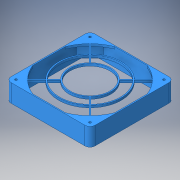
# Autodesk Inventor part: filterFrame
Saved by Autodesk Inventor 2016 (Build 200138000, 138)
## iProperties
Created: 2015-10-01
Part Number: filterFrame
Material: Generic
Document SubType Name: Modeling
Designer: xdlea
Density: 1 g/cm^3
Appearance: Cyan
fanCenter: 2.205 in
d39: 0.059 in
Author: xdlea
Autodesk Inventor part; units mm, degrees
ref_plane "YZ Plane" through (0, 0, 0) normal (1, 0, 0) x (0, 1, 0)
ref_plane "XZ Plane" through (0, 0, 0) normal (0, 1, 0) x (-1, 0, 0)
ref_plane "XY Plane" through (0, 0, 0) normal (0, 0, 1) x (1, 0, 0)
sketch "Sketch1" plane through (0, 0, 0) normal (0, 1, 0) x (-1, 0, 0)
  line L0 (-59.5, 59.5) -> (59.5, 59.5)
  line L1 (59.5, 59.5) -> (59.5, -59.5)
  line L2 (59.5, -59.5) -> (-59.5, -59.5)
  line L3 (-59.5, -59.5) -> (-59.5, 59.5)
  line L4 (-59.5, 59.5) -> (59.5, -59.5) construction
  line L5 (59.5, 59.5) -> (-59.5, -59.5) construction
  circle A0 centre (52.4, 52.4) radius 1.5
  circle A1 centre (52.4, -52.4) radius 1.5
  arc A2 (58, 23.2863) -> (23.2863, 58) centre (0, 0) ccw
  arc A3 (23.2863, -58) -> (58, -23.2863) centre (0, 0) ccw
  arc A4 (-58, -23.2863) -> (-23.2863, -58) centre (0, 0) ccw
  arc A5 (-23.2863, 58) -> (-58, 23.2863) centre (0, 0) ccw
  line L6 (23.2863, 58) -> (-23.2863, 58)
  line L7 (-58, 23.2863) -> (-58, -23.2863)
  line L8 (-23.2863, -58) -> (23.2863, -58)
  line L9 (58, -23.2863) -> (58, 23.2863)
  arc A6 (59.5, 52.4) -> (52.4, 59.5) centre (52.4, 52.4) ccw
  line L10 (48.2954, 59.5) -> (44.1942, 44.1942)
  line L11 (44.1942, 44.1942) -> (59.5, 48.2954)
  circle A7 centre (0, 0) radius 28
  circle A8 centre (0, 0) radius 29.5
  line L12 (44.7213, 43.6607) -> (21.3832, 20.3226)
  line L13 (20.3226, 21.3832) -> (43.6607, 44.7213)
  circle A9 centre (0, 0) radius 43.6607 construction
  line L14 (44.7213, 43.6607) -> (0, 43.6607) construction
  circle A10 centre (0, 0) radius 44.4107
  circle A11 centre (0, 0) radius 42.9107
  point P0 (0, 58)
  dimension "d0" = 119
  dimension "d1" = 3
  dimension "d2" = 104.8
  dimension "d4" = 62.5
  dimension "d7" = 116
  dimension "d9" = 30
  dimension "d38" = 56
  dimension "d39" = 1.5
  dimension "d40" = 1.5
  dimension "d41" = 1.5
  dimension "d83" = 1.5
  dimension "d84" = 0.75
  constraints: 30 end point, 16 point on circle, 11 centre point, 8 coincident, 7 parallel, 6 point on line, 5 equal length, 4 equal radius, 4 vertical alignment, 3 horizontal, 3 midpoint, 2 perpendicular, 2 tangent, 1 horizontal alignment, 3 other
  measures "d0" distance of L0.end L1.end
  measures "d1" diameter of A0
  measures "d2" distance of A1.centre A0.centre
  measures "d4" radius of A2
  measures "d7" distance between parallel lines of L8 L6
  measures "d9" angle of L5 L10
  measures "d38" diameter of A7
  measures "d39" distance between parallel lines of L8 L2
  measures "d40" radial gap between concentric circles of A8 A7
  measures "d41" distance between parallel lines of L12 L13
  measures "d83" radial gap between concentric circles of A11 A10
extrude "Extrusion8" add sketch "Sketch1" along normal blind 3.175 contours L0 L10 L11 L1 L2 L3 | L0 A6 L1 L11 L10 | L0 L1 A6 | A8 | A0 | A1
extrude "Extrusion9" add sketch "Sketch1" along normal blind 3.175 contours A2 L12 A10 L13 | L12 A11 L13 A10 | L12 A8 L13 A11 picked at (31.1052, 30.2803) picked at (23.6041, 24.429)
extrude "Extrusion10" cut sketch "Sketch1" along normal up to next contours L0 L1 A6 | A0
pattern_circular "Circular Pattern4" count 4 over 360 about axis through (0, 0, 0) along (0, 1, 0) of "Extrusion10", "Extrusion9"
sketch "Sketch4" plane through (0, 0, 0) normal (0, -1, 0) x (1, 0, 0)
  arc A0 (-52.4, 59.5) -> (-59.5, 52.4) centre (-52.4, 52.4) ccw projected
  line L0 (-52.4, 59.5) -> (52.4, 59.5) projected
  line L1 (-59.5, -52.4) -> (-59.5, 52.4) projected
  arc A1 (-59.5, -52.4) -> (-52.4, -59.5) centre (-52.4, -52.4) ccw projected
  line L2 (52.4, -59.5) -> (-52.4, -59.5) projected
  arc A2 (52.4, -59.5) -> (59.5, -52.4) centre (52.4, -52.4) ccw projected
  line L3 (59.5, 52.4) -> (59.5, -52.4) projected
  arc A3 (59.5, 52.4) -> (52.4, 59.5) centre (52.4, 52.4) ccw projected
  line L4 (52.4, 58) -> (-52.4, 58)
  arc A4 (-52.4, 58) -> (-58, 52.4) centre (-52.4, 52.4) ccw
  line L5 (-58, 52.4) -> (-58, -52.4)
  arc A5 (-58, -52.4) -> (-52.4, -58) centre (-52.4, -52.4) ccw
  line L6 (-52.4, -58) -> (52.4, -58)
  arc A6 (52.4, -58) -> (58, -52.4) centre (52.4, -52.4) ccw
  line L7 (58, -52.4) -> (58, 52.4)
  arc A7 (58, 52.4) -> (52.4, 58) centre (52.4, 52.4) ccw
  line L8 (-58, 38.8804) -> (-38.8804, 58)
  line L9 (-52.4, 52.4) -> (-48.4402, 48.4402) construction
  line L10 (-52.4, 52.4) -> (-56.3598, 56.3598) construction
  circle A8 centre (-52.4, 52.4) radius 1.5 projected
  point P0 (0, 0)
  dimension "d51" = 1.5
  dimension "d52" = 45
  constraints: 14 end point, 9 point on circle, 4 centre point, 2 point on line, 1 collinear, 1 midpoint, 7 other
  measures "d51" distance between parallel lines of L4 L0
  measures "d52" angle of L4 L8
extrude "Extrusion11" add sketch "Sketch4" along normal blind 22.225 contours L0 A3 L3 A2 L2 A1 L1 A0
extrude "Extrusion12" add sketch "Sketch4" along normal blind 19.05 contours L8 L5 A4 L4
pattern_circular "Circular Pattern5" count 4 over 360 about axis through (0, 0, 0) along (0, 1, 0) of "Extrusion12"
extrude "Extrusion18" add sketch "Sketch1" along normal blind 3.175 contours A10 L13 A11 L12 | L12 A11 L13 A10
equation "\"d0\" = length"
equation "\"d1\" = holeSize"
equation "\"d2\" = dHoles"
equation "\"d4\" = 0.5 * fanDia"
equation "\"d7\" = fanCutOff"
equation "\"d38\" = fanCenter"
equation "\"d40\" = d39"
equation "\"d41\" = d40"
equation "\"d83\" = d39"
equation "\"d84\" = 0.5 * d39"
equation "\"d51\" = d40"
equation "\"d55\" = filterHeight"
equation "\"holeSize\" = 3"
equation "\"filterHeight\" = 19.05"
equation "\"length\" = 119"
equation "\"dHoles\" = 104.8"
equation "\"fanDia\" = 125"
equation "\"fanCutOff\" = 116"
equation "\"fanCenter\" = 56"
body "Solid3"
